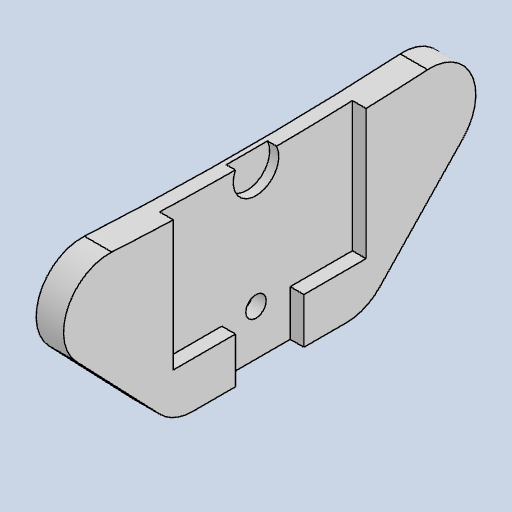
# Autodesk Inventor part: base_cover
Saved by Autodesk Inventor 2026.3 (Build 303398000, 398)
## iProperties
Created: 2026-06-06
Part Number: base_cover
Material: Generic
Document SubType Name: Modeling
Designer: gakut
Density: 1 g/cm^3
Appearance: Default
Author: gakut
## iProperties of the stored document base_cover_3DPrint.ipt
Created: 2026-06-06
Part Number: base_cover_3DPrint
Material: Generic
Document SubType Name: Modeling
Designer: gakut
Density: 1 g/cm^3
Appearance: Default
Author: gakut
Autodesk Inventor part; units mm, degrees
ref_plane "YZ Plane" through (0, 0, 0) normal (1, 0, 0) x (0, 1, 0)
ref_plane "XZ Plane" through (0, 0, 0) normal (0, 1, 0) x (-1, 0, 0)
ref_plane "XY Plane" through (0, 0, 0) normal (0, 0, 1) x (1, 0, 0)
sketch "Sketch1" plane through (0, 0, 0) normal (1, 0, 0) x (0, 1, 0)
  line L0 (10, 21.125) -> (-10, 21.125)
  line L1 (-10, 21.125) -> (-10, -21.125)
  line L2 (-10, -21.125) -> (10, -21.125)
  line L3 (10, -21.125) -> (10, 21.125)
  line L4 (10, 21.125) -> (-10, -21.125) construction
  line L5 (-10, 21.125) -> (10, -21.125) construction
  point P0 (0, 0)
  dimension "d0" = 42.25
  dimension "d1" = 20
  constraints: 12 end point, 2 midpoint, 2 parallel, 1 horizontal, 1 perpendicular
  measures "d0" distance of L0.end L1.end
  measures "d1" distance of L1.end L2.end
extrude "Extrusion1" add sketch "Sketch1" along normal blind 6
sketch "Sketch2" plane through (6, 0, 0) normal (1, 0, 0) x (0, 0, -1)
  line L0 (-21.125, 0) -> (-7.5, 0)
  line L1 (-7.5, 0) -> (-7.5, -10)
  line L2 (-21.125, -10) -> (21.125, -10) projected
  line L3 (7.5, 0) -> (21.125, 0)
  line L4 (21.125, -10) -> (21.125, 10) projected
  line L5 (7.5, 0) -> (7.5, -10.6285)
  line L6 (-21.125, -10) -> (21.125, -10) projected
  line L7 (21.125, -10) -> (21.125, 10) projected
  line L8 (21.125, 10) -> (-21.125, 10) projected
  line L9 (-21.125, 10) -> (-21.125, -10) projected
  point P0 (0, 0)
  point P1 (0, -10)
  point P2 (-21.125, 0)
  point P3 (7.5, -10)
  dimension "d4" = 15
  dimension "d6" = 10
  dimension "d7" = 7.5
  constraints: 8 end point, 3 point on line, 2 midpoint, 1 horizontal, 1 perpendicular, 1 vertical
  measures "d4" distance between parallel lines of L5 L1
  measures "d6" distance of L0.end L1.end
  measures "d7" distance from line of point (0, -10) L1
extrude "Extrusion2" cut sketch "Sketch2" against normal blind 3 contours L9 L8 L4 L3 L5 L2 L1 L0
sketch "Sketch4" plane through (0, 0, 0) normal (-1, 0, 0) x (0, 0, 1)
  arc A0 (21.125, 28.5) -> (190.4596, 58.7605) centre (0, 635.6334) ccw projected
  circle A1 centre (0, 635.6334) radius 607.5008
  circle A2 centre (0, 635.6334) radius 607.5008
  circle A3 centre (0, 635.6334) radius 617.5008
  line L0 (21.125, 0) -> (21.125, -10) projected
  line L1 (21.125, -10) -> (50, 20.1602)
  line L2 (-7.5, -10) -> (-21.125, -10) projected
  line L3 (-21.125, -10) -> (-50, 20.1602)
  line L4 (-50, 20.1602) -> (-50, 30.1937)
  line L5 (50, 20.1602) -> (50, 30.1937)
  line L6 (21.125, -10) -> (-21.125, -10) projected
  point P0 (0, 0)
  dimension "d17" = 0
  dimension "d18" = 10
  dimension "d19" = 100
  constraints: 8 end point, 6 point on circle, 3 centre point, 1 horizontal alignment, 1 perpendicular, 1 vertical, 1 vertical alignment
  measures "d17" radial gap between concentric circles of A1 A2
  measures "d18" radial gap between concentric circles of A2 A3
  measures "d19" distance of L1.end L3.end
extrude "Extrusion3" add sketch "Sketch4" against normal blind 3 contours A0 L5 A3 L4 A1 | L1 L6 L2 L3 A3 picked at (-31.0009, 22.4071)
fillet "Fillet1" radius 10 4 edges at (1.5, 20.1602, 50) (1.5, 20.1602, -50) (1.5, 30.1937, -50) (1.5, 30.1937, 50)
sketch "Sketch3" plane through (3, 0, 0) normal (1, 0, 0) x (0, 0, -1)
  point P0 (0, 0)
  point P1 (0, 0)
  point P2 (7.5, 0)
  constraints: 1 coincident, 1 horizontal alignment
hole "Hole1" at (3, 0, 0) direction (-1, 0, 0) diameter 4.5 end through all
sketch "Sketch5" plane through (3, 0, 0) normal (1, 0, 0) x (0, 0, -1)
  line L0 (-21.125, -10) -> (-7.5, -10) projected
  line L1 (-21.125, -10) -> (21.125, -10)
  line L2 (21.125, -10) -> (21.125, 40)
  line L3 (21.125, 40) -> (-21.125, 40)
  line L4 (-21.125, 40) -> (-21.125, -10)
  arc A0 (-34.605, 29.119) -> (-42.3979, 12.2197) centre (-35.1746, 19.1352) ccw projected
  line L5 (-42.3979, 12.2197) -> (-21.125, -10) projected
  line L6 (-21.125, 0) -> (-21.125, -10) projected
  line L7 (-7.5, 0) -> (-21.125, 0) projected
  line L8 (-7.5, -10) -> (-7.5, 0) projected
  line L9 (7.5, -10) -> (-7.5, -10) projected
  line L10 (7.5, 0) -> (7.5, -10) projected
  line L11 (21.125, 0) -> (7.5, 0) projected
  line L12 (21.125, -10) -> (21.125, 0) projected
  line L13 (21.125, -10) -> (42.3979, 12.2197) projected
  arc A1 (42.3979, 12.2197) -> (34.605, 29.119) centre (35.1746, 19.1352) ccw projected
  arc A2 (-34.605, 29.119) -> (34.605, 29.119) centre (0, 635.6334) ccw projected
  circle A3 centre (0, 0) radius 2.25 projected
  point P0 (21.125, 28.5)
  point P1 (-21.125, 28.5)
  dimension "d26" = 50
  constraints: 8 end point, 2 parallel, 1 horizontal, 1 perpendicular, 1 vertical alignment
  measures "d26" distance between parallel lines of L9 L3
extrude "Extrusion4" add sketch "Sketch5" along normal up to surface (3 mm away) contours L5 A0 A2 L4 | L2 A2 A1 L13
sketch "Sketch6" plane through (3, 0, 0) normal (1, 0, 0) x (0, 0, -1)
  circle A0 centre (0, 26) radius 5
  point P0 (0, 0)
  dimension "d27" = 26
  dimension "d28" = 10
  constraints: 1 centre point, 1 vertical alignment
  measures "d27" distance of point (0, 0) A0.centre
  measures "d28" diameter of A0
extrude "Extrusion5" cut sketch "Sketch6" against normal blind 2
fillet "Fillet2" radius 10 2 edges at (3, -10, -21.125) (3, -10, 21.125)
equation "\"d7\" = 0.5 * d4"
body "Solid1"
